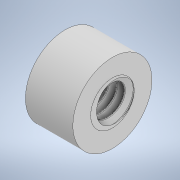
# Autodesk Inventor part: cap
Saved by Autodesk Inventor 2020 (Build 240168000, 168)
## iProperties
Created: 2020-05-22
Part Number: cap
Material: Generic
Document SubType Name: Modeling
Designer: alejandrosalazar
Density: 1 g/cm^3
Appearance: Default
Author: alejandrosalazar
Autodesk Inventor part; units mm, degrees
ref_plane "YZ Plane" through (0, 0, 0) normal (1, 0, 0) x (0, 1, 0)
ref_plane "XZ Plane" through (0, 0, 0) normal (0, 1, 0) x (-1, 0, 0)
ref_plane "XY Plane" through (0, 0, 0) normal (0, 0, 1) x (1, 0, 0)
sketch "Sketch1" plane through (0, 0, 0) normal (1, 0, 0) x (0, 1, 0)
  circle A0 centre (0, 0) radius 5
  dimension "d0" = 10
  constraints: 1 centre point, 1 coincident
  measures "d0" diameter of A0
extrude "Extrusion1" add sketch "Sketch1" along normal blind 6
sketch "Sketch2" plane through (6, 0, 0) normal (1, 0, 0) x (0, 0, -1)
  circle A0 centre (0, 0) radius 2.75
  dimension "d3" = 5.5
  constraints: 1 centre point, 1 coincident
  measures "d3" diameter of A0
extrude "Extrusion2" cut sketch "Sketch2" against normal blind 3
sketch "Sketch15" plane through (6, 0, 0) normal (0, -1, 0) x (0, 0, 1)
  line L0 (2.75, 0) -> (2.75, 3)
  line L1 (2.75, 3) -> (2.0085, 3)
  line L2 (2.0085, 3) -> (2.0085, 0)
  line L3 (2.0085, 0) -> (2.75, 0)
  line L4 (0, -2.5086) -> (0, 7.4181) projected
  constraints: 8 end point
revolve "Revolution6" add sketch "Sketch15" angle 360 about axis through (6, 0, 0) along (-1, 0, 0) separate body
sketch "Sketch14" plane through (6, 0, 2.75) normal (0, 1, 0) x (-1, 0, 0)
  line L0 (-0.5834, -0.0507) -> (-0.5001, -0.0507) construction
  line L1 (0.0832, -0.6911) -> (-0.0001, -0.8511) construction
  line L2 (-1.0001, -0.8511) -> (-1.0834, -0.6911) construction
  line L3 (-0.4168, -0.0507) -> (-0.5001, 0.1093) construction
  line L4 (-0.5001, 0.1093) -> (-0.5834, -0.0507) construction
  line L5 (-1.0001, -0.8511) -> (-0.9168, -0.6911) construction
  line L6 (-0.4168, -0.0507) -> (-0.0834, -0.6911)
  line L7 (-1.0834, -0.6911) -> (-0.9168, -0.6911) construction
  arc A0 (-1.0834, -0.6911) -> (-1.0001, -0.7416) centre (-1.0001, -0.6477) ccw construction
  line L8 (0.0832, -0.6911) -> (-0.0834, -0.6911) construction
  line L9 (-1.0001, -0.8511) -> (-1.0001, -0.6911) construction
  line L10 (-0.0001, -0.8511) -> (-0.0001, -0.6911) construction
  line L11 (-0.5001, 0.1093) -> (-0.5001, -0.0002) construction
  line L12 (-1.0001, -0.7416) -> (-0.0001, -0.7416)
  arc A1 (-1.0001, -0.7416) -> (-0.9168, -0.6911) centre (-1.0001, -0.6477) ccw
  line L13 (-0.0834, -0.6911) -> (-0.0001, -0.8511) construction
  line L14 (-0.9168, -0.6911) -> (-0.5834, -0.0507)
  line L15 (-0.0001, -0.0002) -> (-0.0001, 0.0177)
  line L16 (-0.0001, 0.0177) -> (-0.0001, -0.0002)
  line L17 (-0.0001, -0.0002) -> (0.0334, -0.0002)
  arc A2 (-0.0834, -0.6911) -> (-0.0001, -0.7416) centre (-0.0001, -0.6477) ccw
  arc A3 (-0.0001, -0.7416) -> (0.0832, -0.6911) centre (-0.0001, -0.6477) ccw construction
  arc A4 (-0.5001, -0.0002) -> (-0.5834, -0.0507) centre (-0.5001, -0.0941) ccw
  arc A5 (-0.4168, -0.0507) -> (-0.5001, -0.0002) centre (-0.5001, -0.0941) ccw
  line L18 (-0.5001, -0.0002) -> (-0.5001, -0.0507) construction
  line L19 (-0.5001, -0.0507) -> (-0.4168, -0.0507) construction
  dimension "d110" = 55
  dimension "d111" = 0.1601
  dimension "d112" = 0.1601
  dimension "Sketch14_ThreadOffset" = 0
  dimension "Sketch14_MajorRadius" = 0.7415
  dimension "d115" = 1
  dimension "Sketch14_MinorRadius" = 0
  constraints: 40 end point, 12 point on circle, 10 parallel, 8 tangent, 6 centre point, 6 collinear, 2 midpoint, 2 point on line, 1 horizontal, 1 perpendicular, 3 other
  measures "d110" angle of L6 L14
  measures "d111" distance of L3.end L0.end
  measures "d112" distance of L1.end L10.end
  measures "Sketch14_ThreadOffset" distance between parallel lines of L15 L10
  measures "Sketch14_MajorRadius" distance from line of L12 L15.start
  measures "d115" distance from line of L1.end L9
  measures "Sketch14_MinorRadius" distance edge to line of A5 L17
coil "Coil6" sketch "Sketch14" operation cut axis through (6, 0, 0) along (-1, 0, 0) pitch 1.001 turns 4.995005 hand right bodies 2
equation "\"d110\" = d117"
equation "\"d111\" = 0.160083 * Sketch14_Pitch"
equation "\"d112\" = 0.160083 * Sketch14_Pitch"
equation "\"d115\" = Sketch14_Pitch"
equation "\"d17\" = 55deg"
equation "\"Sketch4_Pitch\" = 0.8"
equation "\"d37\" = 55deg"
equation "\"Sketch6_Pitch\" = 0.5"
equation "\"d57\" = 55deg"
equation "\"Sketch8_Pitch\" = 1"
equation "\"d77\" = 55deg"
equation "\"Sketch10_Pitch\" = 1"
equation "\"d97\" = 55deg"
equation "\"Sketch12_Pitch\" = 1"
equation "\"d117\" = 55deg"
equation "\"Sketch14_Pitch\" = 1"
body "Solid1"
body "Solid7"
